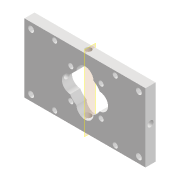
# Autodesk Inventor part: Nikon_Ti2E
Saved by Autodesk Inventor 2022 (Build 260153000, 153)
## iProperties
Created: 2021-06-08
Part Number: Nikon_Ti2E
Material: Generic
Document SubType Name: Modeling
Designer: wanghaoran
Density: 1 g/cm^3
Appearance: Default
Author: wanghaoran
Autodesk Inventor part; units mm, degrees
ref_plane "YZ Plane" through (0, 0, 0) normal (1, 0, 0) x (0, 1, 0)
ref_plane "XZ Plane" through (0, 0, 0) normal (0, 1, 0) x (-1, 0, 0)
ref_plane "XY Plane" through (0, 0, 0) normal (0, 0, 1) x (1, 0, 0)
sketch "Sketch1" plane through (0, 0, 0) normal (0, 0, 1) x (1, 0, 0)
  line L0 (0, 0) -> (120, 0)
  line L1 (120, 0) -> (120, 68)
  line L2 (120, 68) -> (0, 68)
  line L3 (0, 68) -> (0, 0)
  dimension "d0" = 120
  dimension "d1" = 68
  constraints: 8 end point, 2 parallel, 1 horizontal, 1 perpendicular
  measures "d0" distance of L2.end L1.end
  measures "d1" distance of L1.end L0.end
extrude "Extrusion1" add sketch "Sketch1" along normal blind 10
sketch "Sketch2" plane through (0, 0, 10) normal (0, 0, 1) x (1, 0, 0)
  circle A0 centre (6.6, 6) radius 2
  line L0 (0, 0) -> (120, 0) projected
  line L1 (0, 68) -> (0, 0) projected
  circle A1 centre (113.4, 6) radius 2
  circle A2 centre (6.6, 62) radius 2
  circle A3 centre (113.4, 62) radius 2
  circle A4 centre (60, 34) radius 17
  circle A5 centre (45, 49) radius 3.25
  circle A6 centre (75, 49) radius 3.25
  circle A7 centre (45, 19) radius 3.25
  circle A8 centre (75, 19) radius 3.25
  line L2 (120, 68) -> (0, 68) projected
  circle A9 centre (60, 48.4582) radius 8.4721
  circle A10 centre (45.5418, 34) radius 8.4721
  circle A11 centre (60, 19.5418) radius 8.4721
  circle A12 centre (74.4582, 34) radius 8.4721
  point P0 (68.4673, 19.2587)
  point P1 (51.5327, 19.2587)
  point P2 (74.7413, 25.5327)
  point P3 (74.7413, 42.4673)
  point P4 (45.2587, 25.5327)
  point P5 (45.2587, 42.4673)
  point P6 (51.5327, 48.7413)
  point P7 (68.4673, 48.7413)
  dimension "d4" = 4
  dimension "d5" = 6
  dimension "d6" = 6.6
  dimension "d9" = 106.8
  dimension "d12" = 56
  dimension "d15" = 34
  dimension "d16" = 6.5
  dimension "d17" = 15
  dimension "d18" = 15
  dimension "d19" = 34
  dimension "d20" = 60
  dimension "d23" = 30
  dimension "d26" = 30
  dimension "d82" = 360
  constraints: 13 centre point, 2 horizontal, 2 vertical, 21 other
  measures "d4" diameter of A0
  measures "d5" distance from line of L0 A0.centre
  measures "d6" distance from line of L1 A0.centre
  measures "d9" distance of A0.centre A1.centre
  measures "d12" distance of A0.centre A2.centre
  measures "d15" diameter of A4
  measures "d16" diameter of A5
  measures "d17" horizontal distance of A5.centre A4.centre
  measures "d18" horizontal distance of A4.centre A5.centre
  measures "d19" distance from line of L0 A4.centre
  measures "d20" distance from line of L1 A4.centre
  measures "d23" distance of A5.centre A6.centre
  measures "d26" distance of A5.centre A7.centre
extrude "Extrusion2" cut sketch "Sketch2" against normal through all contours A0 | A1 | A2 | A3 | A4 A12 | A4 A12 | A12 A4 A11 A10 A9 | A9 A4 | A4 A9 | A11 A4 | A4 A11 | A10 A4 | A4 A10
sketch "Sketch3" plane through (0, 68, 0) normal (0, 1, 0) x (1, 0, 0)
  circle A0 centre (58.4, -5) radius 2.95
  line L0 (120, 0) -> (0, 0) projected
  line L1 (0, 0) -> (0, -10) projected
  dimension "d33" = 5.9
  dimension "d34" = 5
  dimension "d35" = 58.4
  constraints: 1 centre point
  measures "d33" diameter of A0
  measures "d34" distance from line of L0 A0.centre
  measures "d35" distance from line of L1 A0.centre
extrude "Extrusion3" cut sketch "Sketch3" against normal through all
sketch "Sketch4" plane through (120, 0, 0) normal (1, 0, 0) x (0, 0, -1)
  circle A0 centre (-5, 35) radius 2.95
  line L0 (-10, 0) -> (-10, 68) projected
  line L1 (0, 68) -> (-10, 68) projected
  point P0 (0, 0)
  dimension "d38" = 5.9
  dimension "d39" = 5
  dimension "d40" = 33
  constraints: 1 centre point
  measures "d38" diameter of A0
  measures "d39" horizontal distance of L0 A0.centre
  measures "d40" distance from line of L1 A0.centre
extrude "Extrusion4" cut sketch "Sketch4" against normal through all
sketch "Sketch5" plane through (0, 0, 10) normal (0, 0, 1) x (1, 0, 0)
  circle A0 centre (46, 50) radius 1.35
  circle A1 centre (60, 34) radius 17 projected
  line L0 (46, 50) -> (49.5107, 50)
  line L1 (49.5107, 50) -> (49.5107, 57.375)
  circle A2 centre (76, 50) radius 1.35
  circle A3 centre (46, 20) radius 1.35
  circle A4 centre (76, 20) radius 1.35
  circle A5 centre (30, 64) radius 1.35
  circle A6 centre (90, 64) radius 1.35
  circle A7 centre (30, 4) radius 1.35
  circle A8 centre (90, 4) radius 1.35
  point P0 (0, 0)
  dimension "d43" = 2.7
  dimension "d45" = 14
  dimension "d46" = 16
  dimension "d49" = 30
  dimension "d52" = 30
  dimension "d62" = 2.7
  dimension "d63" = 30
  dimension "d64" = 30
  dimension "d67" = 60
  dimension "d70" = 60
  constraints: 8 centre point, 4 end point, 3 horizontal, 2 vertical, 1 perpendicular, 12 other
  measures "d43" diameter of A0
  measures "d45" horizontal distance of A1.centre L0.start
  measures "d46" vertical distance of L0.start A1.centre
  measures "d49" distance of L0.start A2.centre
  measures "d52" distance of L0.start A3.centre
  measures "d62" diameter of A5
  measures "d63" horizontal distance of A5.centre A1.centre
  measures "d64" horizontal distance of A5.centre A1.centre
  measures "d67" distance of A5.centre A6.centre
  measures "d70" distance of A5.centre A7.centre
hole "Hole1" at (76, 50, 10) at (76, 20, 10) at (46, 20, 10) at (46, 50, 10) at (30, 64, 10) at (90, 64, 10) at (90, 4, 10) at (30, 4, 10) direction (0, 0, -1) diameter 2.8 end through all counterbore diameter 5 counterbore depth 4.9
sketch "Sketch7" plane through (0, 0, 0) normal (0, 0, -1) x (-1, 0, 0)
  circle A0 centre (-113.4, 62) radius 2 projected
  circle A1 centre (-113.4, 6) radius 2 projected
  circle A2 centre (-6.6, 6) radius 2 projected
  circle A3 centre (-6.6, 62) radius 2 projected
  point P0 (0, 0)
hole "Hole2" at (113.4, 62, 0) at (6.6, 62, 0) at (6.6, 6, 0) at (113.4, 6, 0) direction (0, 0, 1) diameter 5.8 end through all counterbore diameter 9.4 counterbore depth 5.4
ref_plane "Work Plane1" through (60, 0, 0) normal (1, 0, 0) x (0, 0, -1)
body "Solid1"
